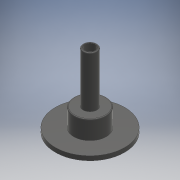
# Autodesk Inventor part: Support
Saved by Autodesk Inventor 2017 (Build 210142000, 142)
## iProperties
Company: FABLAB Frenchmakers
Part Number: Support
Material: Plastique ABS
Document SubType Name: Modeling
Designer: FABLAB Frenchmakers
Density: 1.06 g/cm^3
Appearance: Lisse - Blanc(4)
Mass: 42.9357 g
Surface Area: 175.643 cm^2
Volume: 40.5054 cm^3
Project: 1420 Vauban 3D XL
Catalog Web Link: http://frenchmakers.com/
Stock Number: 1420-03-02
Autodesk Inventor part; units mm, degrees
ref_plane "YZ Plane" through (0, 0, 0) normal (1, 0, 0) x (0, 1, 0)
ref_plane "XZ Plane" through (0, 0, 0) normal (0, 1, 0) x (-1, 0, 0)
ref_plane "XY Plane" through (0, 0, 0) normal (0, 0, 1) x (1, 0, 0)
sketch "Esquisse1" plane through (0, 0, 0) normal (0, 0, 1) x (1, 0, 0)
  circle A0 centre (0, 0) radius 37.5
  dimension "d0" = 75
  constraints: 1 centre point, 1 coincident
  measures "d0" diameter of A0
extrude "Extrusion1" add sketch "Esquisse1" along normal blind 5
sketch "Esquisse2" plane through (0, 0, 5) normal (0, 0, 1) x (1, 0, 0)
  circle A0 centre (0, 0) radius 17.5
  dimension "d3" = 35
  constraints: 1 centre point, 1 coincident
  measures "d3" diameter of A0
extrude "Extrusion2" add sketch "Esquisse2" along normal blind 20
sketch "Esquisse3" plane through (0, 0, 25) normal (0, 0, 1) x (1, 0, 0)
  circle A0 centre (0, 0) radius 7.5
  dimension "d6" = 15
  constraints: 1 centre point, 1 coincident
  measures "d6" diameter of A0
extrude "Extrusion3" add sketch "Esquisse3" along normal blind 55
sketch "Esquisse4" plane through (0, 0, 0) normal (1, 0, 0) x (0, 1, 0)
  line L0 (0, -16) -> (0, 96) projected
  line L1 (-37.5, 0) -> (37.5, 0) projected
  line L2 (-11.225, 0) -> (-11.225, 8.5)
  line L3 (-5.625, 8.5) -> (-5.625, 80)
  line L4 (-7.5, 25) -> (-7.5, 80) projected
  line L5 (-11.225, 0) -> (0, 0)
  line L6 (-5.625, 80) -> (0, 80)
  line L7 (7.5, 80) -> (-7.5, 80) construction
  line L8 (0, 0) -> (0, 80)
  line L9 (-11.225, 8.5) -> (-5.625, 8.5)
  dimension "d9" = 11.25
  dimension "d13" = 22.45
  dimension "d25" = 8.5
  constraints: 12 end point, 3 collinear, 2 perpendicular, 2 point on line, 1 horizontal, 1 parallel
  measures "d9" diameter of L3 L0
  measures "d13" diameter of L2 L0
  measures "d25" distance between parallel lines of L5 L9
revolve "Révolution1" cut sketch "Esquisse4" angle 360 about axis through (0, 0, -10) along (0, 0, 1)
fillet "Congé1" radius 1 2 edges at (-7.5, 0, 80) (-17.5, 0, 25)
chamfer "Chanfrein1" distance 0.5 angle 45 2 edges at (0, 11.225, 0) (-37.5, 0, 0)
chamfer "Chanfrein2" distance 0.25 angle 45 2 edges at (0, 5.625, 80) (0, 5.625, 8.5)
